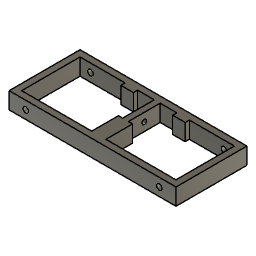
X axis wheel frame v3 (Autodesk Fusion 360 design; units mm, degrees)
Autodesk Fusion 360 part; units mm, degrees
sketch "Sketch1" plane through (0, 0, 0) normal (0, 0, 1) x (1, 0, 0)
  line L0 (80, 0) -> (-80, 0) construction
  line L1 (100, 42.5) -> (-100, 42.5)
  line L2 (-100, 42.5) -> (-100, -42.5)
  line L3 (-100, -42.5) -> (100, -42.5)
  line L4 (100, -42.5) -> (100, 42.5)
  circle A0 centre (80, 0) radius 2.75
  circle A1 centre (-80, 0) radius 2.75
  line L5 (-90, 35) -> (-3.5, 35)
  line L6 (3.5, 35) -> (90, 35)
  line L7 (3.5, -35) -> (90, -35)
  line L8 (-3.5, -35) -> (-90, -35)
  line L9 (-3.5, 35) -> (-3.5, -3)
  line L10 (3.5, -3) -> (3.5, 35)
  line L11 (3.5, -3) -> (8.5, -3)
  line L12 (-3.5, -3) -> (-8.5, -3)
  line L13 (8.5, -3) -> (8.5, -35)
  line L14 (-8.5, -3) -> (-8.5, -35)
  line L15 (-90, 35) -> (-92.5, 35)
  line L16 (-92.5, 35) -> (-92.5, -35)
  line L17 (-92.5, -35) -> (-90, -35)
  line L18 (90, 35) -> (92.5, 35)
  line L19 (92.5, 35) -> (92.5, -35)
  line L20 (92.5, -35) -> (90, -35)
  line L21 (-23.5, 35) -> (-23.5, 30)
  line L22 (-23.5, 30) -> (-38.5, 30)
  line L23 (-38.5, 30) -> (-38.5, 35)
  line L24 (23.5, 35) -> (23.5, 30)
  line L25 (23.5, 30) -> (38.5, 30)
  line L26 (38.5, 30) -> (38.5, 35)
  dimension "d9" = 160
  dimension "d12" = 200
  dimension "d13" = 85
  dimension "d14" = 5.5
  dimension "d15" = 5.5
  dimension "d46" = 7
  dimension "d47" = 38
  dimension "d55" = 5
  dimension "d56" = 5
  dimension "d66" = 2.5
  dimension "d67" = 2.5
  dimension "d68" = 20
  dimension "d69" = 15
  dimension "d70" = 20
  dimension "d71" = 15
  constraint horizontal L1
  constraint vertical L2
  constraint horizontal L3
  constraint vertical L4
  constraint coincident L0.start A0.centre
  constraint coincident L0.end A1.centre
  constraint vertical L9
  constraint vertical L10
  constraint perpendicular L10 L11
  constraint coincident L7 L13.end
  constraint perpendicular L7 L13
  constraint coincident L8 L14.end
  constraint perpendicular L8 L14
  constraint perpendicular L5 L16
  constraint perpendicular L18 L19
  constraint coincident L5 L21.start
  constraint perpendicular L21 L22
  constraint coincident L5 L23.end
  constraint perpendicular L5 L23
  constraint perpendicular L24 L25
  constraint coincident L6 L26.end
  constraint perpendicular L6 L26
  measures "d9" distance of L0.start L0.end
  measures "d12" distance of L1.start L1.end
  measures "d13" distance of L1.start L3.end
  measures "d14" diameter of A0
  measures "d15" diameter of A1
  measures "d46" distance of L6.start L5.end
  measures "d47" distance of L6.start L10.start
  measures "d55" distance of L10.start L11.end
  measures "d56" distance of L9.end L12.end
  measures "d66" distance of L5.start L15.end
  measures "d67" distance of L6.end L18.end
  measures "d68" distance of L5.end L21.start
  measures "d69" distance of L21.end L22.end
  measures "d70" distance of L6.start L24.start
  measures "d71" distance of L24.end L25.end
sketch "Sketch3" plane through (0, -42.5, 0) normal (0, -1, 0) x (1, 0, 0)
  line L0 (-100, 0) -> (100, 0)
  line L1 (100, 0) -> (100, 20)
  line L2 (100, 20) -> (-100, 20)
  line L3 (-100, 20) -> (-100, 0)
  line L4 (-100, 10) -> (-80, 10) construction
  line L5 (100, 10) -> (80, 10) construction
  dimension "d50" = 20
  dimension "d51" = 20
  constraint midpoint L3 L4.start
  constraint perpendicular L3 L4
  constraint midpoint L1 L5.start
  constraint perpendicular L1 L5
  measures "d50" distance of L4.start L4.end
  measures "d51" distance of L5.start L5.end
sketch "Sketch4" plane through (-3.5, 0, 0) normal (-1, 0, 0) x (0, -1, 0)
  line L0 (-35, 0) -> (3, 0)
  line L1 (3, 0) -> (3, 20)
  line L2 (3, 20) -> (-35, 20)
  line L3 (-35, 20) -> (-35, 0)
  line L4 (-35, 10) -> (3, 10) construction
  line L5 (-16, 20) -> (-16, 0) construction
  circle A0 centre (-16, 10) radius 2.75
  dimension "d62" = 5.5
  constraint midpoint L3 L4.start
  constraint midpoint L1 L4.end
  constraint midpoint L2 L5.start
  constraint midpoint L0 L5.end
  constraint midpoint L4 A0.centre
  measures "d62" diameter of A0
extrude "Extrude7" add sketch "Sketch1" along normal blind 20 contours L1 L2 L3 L4 | L5 L21 L22 L23 | L6 L24 L25 L26
hole "Hole6" at (-80, -42.5, 10) at (80, -42.5, 10) direction (0, 1, 0) diameter 6.6 depth 85 tip angle 180
hole "Hole7" at (-3.5, 16, 10) direction (1, 0, 0) diameter 5.5 depth 7 tip angle 180
